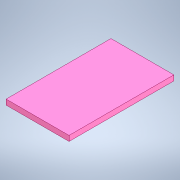
# Autodesk Inventor part: Roller Base
Saved by Autodesk Inventor 2022.4 (Build 264492000, 492)
## iProperties
Created: 2024-02-15
Part Number: Roller Base
Material: Generic
Document SubType Name: Modeling
Designer: t60147996
Density: 1 g/cm^3
Appearance: Pink
Author: t60147996
Autodesk Inventor part; units mm, degrees
ref_plane "YZ Plane" through (0, 0, 0) normal (1, 0, 0) x (0, 1, 0)
ref_plane "XZ Plane" through (0, 0, 0) normal (0, 1, 0) x (-1, 0, 0)
ref_plane "XY Plane" through (0, 0, 0) normal (0, 0, 1) x (1, 0, 0)
sketch "Sketch1" plane through (0, 0, 0) normal (0, 1, 0) x (-1, 0, 0)
  line L0 (76.2, 127) -> (-76.2, 127)
  line L1 (-76.2, 127) -> (-76.2, -127)
  line L2 (-76.2, -127) -> (76.2, -127)
  line L3 (76.2, -127) -> (76.2, 127)
  line L4 (76.2, 127) -> (-76.2, -127) construction
  line L5 (-76.2, 127) -> (76.2, -127) construction
  point P0 (0, 0)
  dimension "d0" = 152.4
  dimension "d1" = 254
  constraints: 12 end point, 2 midpoint, 2 parallel, 1 horizontal, 1 perpendicular
  measures "d0" distance of L2.end L1.end
  measures "d1" distance of L1.end L0.end
extrude "Extrusion1" add sketch "Sketch1" along normal blind 12.7
body "Solid1"
